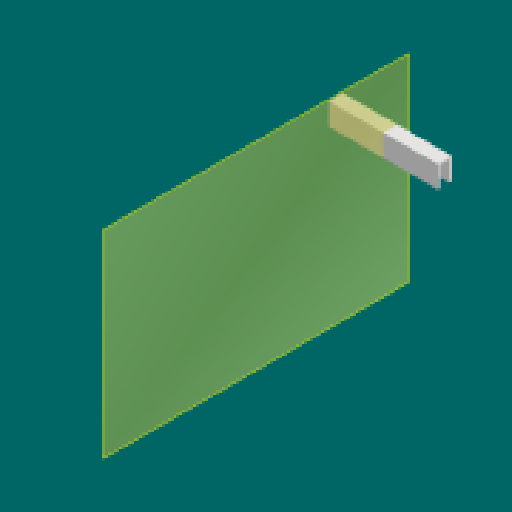
# Autodesk Inventor part: servo_mount
Saved by Autodesk Inventor 2023 (Build 270158000, 158)
## iProperties
Created: 2022-11-12
Part Number: servo_mount
Material: Generic
Document SubType Name: Modeling
Designer: sgodi
Density: 1 g/cm^3
Appearance: Default
Author: sgodi
Autodesk Inventor part; units mm, degrees
ref_plane "YZ Plane" through (0, 0, 0) normal (1, 0, 0) x (0, 1, 0)
ref_plane "XZ Plane" through (0, 0, 0) normal (0, 1, 0) x (-1, 0, 0)
ref_plane "XY Plane" through (0, 0, 0) normal (0, 0, 1) x (1, 0, 0)
ref_plane "Work Plane1" through (0, 0, 0) normal (1, 0, 0) x (0, 1, 0)
sketch "Sketch1" plane through (0, 0, 0) normal (1, 0, 0) x (0, 1, 0)
  line L0 (0, -147.65) -> (139.61, -147.65) projected
  line L1 (-10, -157.65) -> (139.61, -157.65) projected
  line L2 (147.11, -144.65) -> (129.61, -144.65)
  line L3 (129.61, -144.65) -> (129.61, -160.65)
  line L4 (129.61, -160.65) -> (147.11, -160.65)
  line L5 (147.11, -160.65) -> (147.11, -144.65)
  line L6 (139.61, 157.65) -> (139.61, -157.65) projected
  line L7 (129.61, -144.65) -> (139.61, -144.65)
  line L8 (139.61, -144.65) -> (139.61, -147.65)
  line L9 (139.61, -147.65) -> (129.61, -147.65)
  line L10 (129.61, -147.65) -> (129.61, -144.65)
  line L11 (129.61, -160.65) -> (139.61, -160.65)
  line L12 (139.61, -160.65) -> (139.61, -157.65)
  line L13 (139.61, -157.65) -> (129.61, -157.65)
  line L14 (129.61, -157.65) -> (129.61, -160.65)
  line L15 (139.61, -147.65) -> (147.11, -147.65)
  point P0 (0, 0)
  point P1 (138.36, -144.65)
  dimension "d0" = 3
  dimension "d1" = 3
  dimension "d2" = 7.5
  dimension "d3" = 17.5
  constraints: 26 end point, 6 parallel, 3 horizontal, 3 perpendicular, 2 point on line, 1 midpoint
  measures "d0" distance from line of point (138.36, -144.65) L0
  measures "d1" distance between parallel lines of L4 L1
  measures "d2" distance between parallel lines of L6 L5
  measures "d3" distance of L3.end L4.end
extrude "Extrusion1" add sketch "Sketch1" along normal mid plane 123.8834 contours L15 L5 L4 L12 L6 | L1 L12 L4 L3
ref_plane "Work Plane2" through (-75.2, 139.61, -157.65) normal (0, 1, 0) x (0, 0, 1)
sketch "Sketch2" plane through (-61.9417, 147.11, -147.65) normal (0, 1, 0) x (1, 0, 0)
  line L0 (0, 0) -> (123.8834, 0) projected
  line L1 (0, 13) -> (123.8834, 13) projected
  line L2 (10, 0) -> (113.8834, 0)
  line L3 (113.8834, 0) -> (113.8834, 13)
  line L4 (113.8834, 13) -> (10, 13)
  line L5 (10, 13) -> (10, 0)
  line L6 (123.8834, 13) -> (123.8834, 0) projected
  line L7 (0, 0) -> (0, 13) projected
  point P0 (61.9417, -147.65)
  point P1 (123.8834, 6.5)
  point P2 (10, 13)
  dimension "d6" = 123.8834
  dimension "d10" = 10
  dimension "d11" = 10
  constraints: 8 end point, 2 parallel, 2 point on line, 1 horizontal, 1 midpoint, 1 perpendicular
  measures "d6" distance of L1.start L1.end
  measures "d10" distance from line of point (123.883, 6.5) L3
  measures "d11" distance between parallel lines of L7 L5
extrude "Extrusion2" cut sketch "Sketch2" against normal up to surface (7.5 mm away) contours L5 L1 L3 L0
sketch "Sketch4" plane through (61.9417, 129.61, -160.65) normal (0, 0, -1) x (-1, 0, 0)
  line L0 (10, 10) -> (0, 10) projected
  line L1 (0, 17.5) -> (0, 10) projected
  line L2 (10, 10) -> (0, 17.5) construction
  line L3 (10, 17.5) -> (10, 10) projected
  line L4 (0, 10) -> (10, 17.5) construction
  line L5 (123.8834, 10) -> (113.8834, 10) projected
  line L6 (123.8834, 17.5) -> (113.8834, 17.5) projected
  line L7 (113.8834, 10) -> (123.8834, 17.5) construction
  line L8 (123.8834, 0) -> (123.8834, 10) projected
  line L9 (113.8834, 17.5) -> (123.8834, 10) construction
  circle A0 centre (5, 13.75) radius 1.524
  circle A1 centre (118.8834, 13.75) radius 1.524
  line L10 (123.8834, 0) -> (0, 0) projected
  circle A2 centre (5, 5) radius 1.524
  circle A3 centre (118.8834, 5) radius 1.524
  point P0 (61.9417, -129.61)
  dimension "d18" = 3.048
  dimension "d19" = 3.048
  dimension "d20" = 5
  dimension "d21" = 3.048
  dimension "d22" = 3.048
  constraints: 8 end point, 4 centre point, 4 coincident, 3 midpoint, 2 vertical alignment, 1 horizontal alignment
  measures "d18" diameter of A0
  measures "d19" diameter of A1
  measures "d20" distance from line of L10 point (5, 5)
  measures "d21" diameter of A2
  measures "d22" diameter of A3
extrude "Extrusion4" cut sketch "Sketch4" against normal up to next
sketch "Sketch5" plane through (61.9417, 129.61, -160.65) normal (0, 0, -1) x (-1, 0, 0)
  line L0 (17.4917, 6) -> (106.3917, 6)
  line L1 (106.3917, 6) -> (106.3917, 0)
  line L2 (106.3917, 0) -> (17.4917, 0)
  line L3 (17.4917, 0) -> (17.4917, 6)
  line L4 (123.8834, 0) -> (0, 0) projected
  line L5 (0, 0) -> (0, 17.5) projected
  line L6 (17.4917, 6) -> (10, 0)
  line L7 (123.8834, 0) -> (0, 0) projected
  line L8 (106.3917, 6) -> (113.8834, 0)
  point P0 (61.9417, -129.61)
  point P1 (113.8834, 10)
  point P2 (10, 10)
  point P3 (17.4917, 0)
  point P4 (106.3917, 0)
  dimension "d25" = 88.9
  dimension "d26" = 6
  dimension "d27" = 123.8834
  dimension "d28" = 17.4917
  constraints: 12 end point, 2 parallel, 2 point on line, 2 vertical alignment, 1 collinear, 1 horizontal, 1 perpendicular
  measures "d25" distance of L0.start L0.end
  measures "d26" distance between parallel lines of L2 L0
  measures "d27" distance of L4.start L4.end
  measures "d28" distance between parallel lines of L5 L3
extrude "Extrusion5" cut sketch "Sketch5" against normal up to next
fillet "Fillet1" radius 3.175 12 edges at (44.45, 135.61, -159.15) (-44.45, 135.61, -159.15) (-51.9417, 129.61, -159.15) (-61.9417, 129.61, -159.15) (51.9417, 129.61, -159.15) (61.9417, 129.61, -159.15) (51.9417, 139.61, -159.15) (51.9417, 147.11, -154.15) (61.9417, 147.11, -154.15) (-61.9417, 147.11, -154.15) (-51.9417, 147.11, -154.15) (-51.9417, 139.61, -159.15)
equation "\"d1\" = d0"
equation "\"d11\" = d10"
equation "\"d28\" = -0.5 * d25 + 0.5 * d27"
